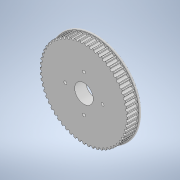
# Autodesk Inventor part: プーリ_歯数60_3Dプリンタ
Saved by Autodesk Inventor 2021 (Build 250183000, 183)
## iProperties
Created: 2022-02-13
Part Number: プーリ_歯数60_3Dプリンタ
Material: 一般
Document SubType Name: Modeling
Designer: hirohumi
Density: 1 g/cm^3
Appearance: 既定
Author: hirohumi
Autodesk Inventor part; units mm, degrees
ref_plane "YZ Plane" through (0, 0, 0) normal (1, 0, 0) x (0, 1, 0)
ref_plane "XZ Plane" through (0, 0, 0) normal (0, 1, 0) x (-1, 0, 0)
ref_plane "XY Plane" through (0, 0, 0) normal (0, 0, 1) x (1, 0, 0)
sketch "スケッチ1" plane through (0, 0, 0) normal (0, 0, 1) x (1, 0, 0)
  arc A0 (11.2031, 43.8361) -> (-12.7392, 43.4146) centre (0, 0) ccw construction
  arc A1 (-0.569, 47.1716) -> (-1.072, 46.6316) centre (-0.5629, 46.6616) ccw
  arc A2 (1.072, 46.6316) -> (0.569, 47.1716) centre (0.5629, 46.6616) ccw
  arc A3 (-2.3679, 45.183) -> (-1.072, 46.6316) centre (-2.4396, 46.5511) ccw
  arc A4 (1.072, 46.6316) -> (2.3679, 45.183) centre (2.4396, 46.5511) ccw
  arc A5 (0.569, 47.1716) -> (-0.569, 47.1716) centre (0, 0) ccw
  line L0 (-2.3679, 45.183) -> (0, 0)
  line L1 (0, 0) -> (2.3679, 45.183)
  line L2 (0, 0) -> (0, 8.5337) construction
  dimension "d0" = 0.51
  dimension "d1" = 0.51
  dimension "d2" = 1.37
  dimension "d3" = 1.37
  dimension "d4" = 6
  dimension "d5" = 3
  dimension "d6" = 47.175
  dimension "d7" = 1.93
  constraints: 14 point on circle, 6 centre point, 6 end point, 6 tangent, 2 coincident, 1 vertical
  measures "d0" radius of A1
  measures "d1" radius of A2
  measures "d2" radius of A3
  measures "d3" radius of A4
  measures "d4" angle of L1 L0
  measures "d5" angle of L2 L0
  measures "d6" radius of A5
  measures "d7" radial gap between concentric circles of A0 A5
extrude "押し出し1" add sketch "スケッチ1" along normal blind 11
pattern_circular "円形状パターン1" count 60 over 360 about axis through (0, 0, 0) along (0, 0, 1) of "押し出し1"
sketch "スケッチ3" plane through (0, 0, 0) normal (0, 0, -1) x (-1, 0, 0)
  circle A0 centre (0, 0) radius 49
  dimension "d16" = 98
  constraints: 1 centre point, 1 coincident
  measures "d16" diameter of A0
extrude "押し出し3" add sketch "スケッチ3" along normal blind 2
fillet "フィレット1" radius 1 2 edges at (49, 0, 0) (49, 0, -2)
sketch "スケッチ4" plane through (0, 0, -2) normal (0, 0, -1) x (-1, 0, 0)
  circle A0 centre (0, 0) radius 10
  circle A1 centre (0, 0) radius 20 construction
  circle A2 centre (0, 20) radius 1.6
  circle A3 centre (-20, 0) radius 1.6
  circle A4 centre (0, -20) radius 1.6
  circle A5 centre (20, 0) radius 1.6
  dimension "d20" = 20
  dimension "d21" = 40
  dimension "d22" = 3.2
  dimension "d23" = 3.2
  dimension "d24" = 3.2
  dimension "d25" = 3.2
  constraints: 6 centre point, 4 point on circle, 3 coincident, 2 horizontal alignment, 2 vertical alignment
  measures "d20" diameter of A0
  measures "d21" diameter of A1
  measures "d22" diameter of A2
  measures "d23" diameter of A3
  measures "d24" diameter of A4
  measures "d25" diameter of A5
extrude "押し出し4" cut sketch "スケッチ4" against normal through all
fillet "フィレット2" radius 1 1 edges at (10, 0, -2)
